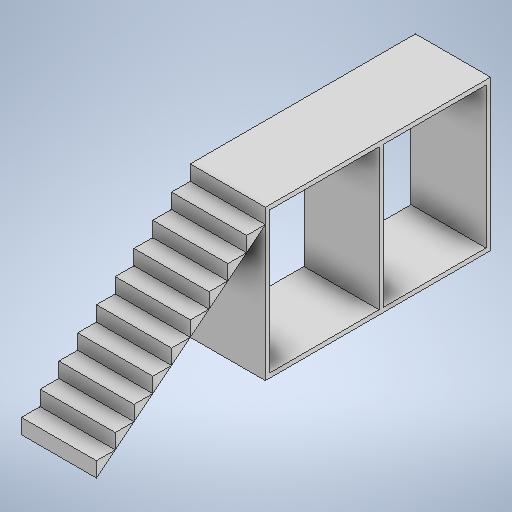
# Autodesk Inventor part: BSH 03 upstairs
Saved by Autodesk Inventor 2025 (Build 290162010, 162A)
## iProperties
Created: 2024-08-27
Part Number: BSH 03 upstairs
Material: Generic
Document SubType Name: Modeling
Designer: DELL
Density: 1 g/cm^3
Appearance: Default
Author: DELL
Autodesk Inventor part; units mm, degrees
ref_plane "YZ Plane" through (0, 0, 0) normal (1, 0, 0) x (0, 1, 0)
ref_plane "XZ Plane" through (0, 0, 0) normal (0, 1, 0) x (-1, 0, 0)
ref_plane "XY Plane" through (0, 0, 0) normal (0, 0, 1) x (1, 0, 0)
sketch "Sketch1" plane through (0, 0, 0) normal (0, 0, 1) x (1, 0, 0)
  line L0 (500, 1500) -> (-500, 1500)
  line L1 (-500, 1500) -> (-500, -1500)
  line L2 (-500, -1500) -> (500, -1500)
  line L3 (500, -1500) -> (500, 1500)
  line L4 (500, 1500) -> (-500, -1500) construction
  line L5 (-500, 1500) -> (500, -1500) construction
  point P0 (0, 0)
  dimension "d0" = 1000
  dimension "d1" = 3000
  constraints: 12 end point, 2 midpoint, 2 parallel, 1 horizontal, 1 perpendicular
  measures "d0" distance of L2.end L1.end
  measures "d1" distance of L1.end L0.end
extrude "Extrusion1" add sketch "Sketch1" along normal blind 2000
sketch "Sketch2" plane through (-500, -1500, 0) normal (-1, 0, 0) x (0, 0, 1)
  line L0 (0, 3000) -> (0, 0) projected
  line L1 (0, 0) -> (2000, 0) projected
  line L2 (2000, 3000) -> (2000, 0) projected
  line L3 (0, 3000) -> (2000, 3000) projected
  line L4 (1800, 0) -> (1800, -250)
  line L5 (1800, -250) -> (1600, -250)
  line L6 (1600, -250) -> (1800, 0)
  point P0 (0, 1500)
  dimension "d4" = 250
  dimension "d5" = 200
  dimension "d6" = 200
  dimension "d7" = 51.34
  constraints: 6 end point, 1 perpendicular, 1 point on line, 1 vertical
  measures "d4" distance of L4.start L4.end
  measures "d5" distance of L4.end L5.end
  measures "d6" distance between parallel lines of L4 L2
  measures "d7" angle of L1 L6
extrude "Extrusion2" add sketch "Sketch2" against normal up to surface (1000 mm away) contours L4 L5 L6
pattern_linear "Rectangular Pattern1" count 9 spacing 320 along (0, -0.7808688, -0.624695) of "Extrusion2"
sketch "Sketch3" plane through (-500, -1500, 0) normal (-1, 0, 0) x (0, 0, 1)
  line L0 (0, 3000) -> (0, 0) projected
  line L1 (0, 0) -> (1800, 0) projected
  line L2 (1800, 0) -> (2000, 0) projected
  line L3 (2000, 3000) -> (2000, 0) projected
  line L4 (0, 3000) -> (2000, 3000) projected
  line L5 (1940, 60) -> (1800, 60)
  line L6 (1800, 60) -> (60, 60)
  line L7 (60, 60) -> (60, 2940)
  line L8 (60, 2940) -> (1940, 2940)
  line L9 (1940, 2940) -> (1940, 60)
  line L10 (1940, 1575.1535) -> (60, 1575.1535)
  line L11 (60, 1575.1535) -> (60, 1515.1535)
  line L12 (60, 1515.1535) -> (1940, 1515.1535)
  line L13 (1940, 1515.1535) -> (1940, 1575.1535)
  point P0 (0, 1500)
  dimension "d13" = 60
  dimension "d14" = 60
  constraints: 18 end point, 2 parallel, 2 point on line, 1 horizontal, 1 perpendicular, 4 other
  measures "d13" distance between parallel lines of L3 L9
  measures "d14" distance between parallel lines of L12 L10
extrude "Extrusion3" cut sketch "Sketch3" against normal through all contours L5 L6 L7 L12 L9 | L10 L7 L8 L9
equation "\"d6\" = d5"
equation "\"d14\" = d13"
body "Solid1"
